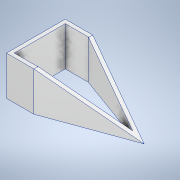
# Autodesk Inventor part: Wedge_wall
Saved by Autodesk Inventor 2020 (Build 240168000, 168)
## iProperties
Created: 2020-01-24
Part Number: Wedge_wall
Material: Aluminum 6061
Document SubType Name: Modeling
Designer: Connor
Density: 2.7 g/cm^3
Appearance: Aluminum - Flat
Mass: 1317.92 g
Surface Area: 1114.86 cm^2
Volume: 488.119 cm^3
Author: Connor
Autodesk Inventor part; units mm, degrees
ref_plane "YZ Plane" through (0, 0, 0) normal (1, 0, 0) x (0, 1, 0)
ref_plane "XZ Plane" through (0, 0, 0) normal (0, 1, 0) x (-1, 0, 0)
sketch "Sketch2" plane through (0, 0, 0) normal (0, 1, 0) x (-1, 0, 0)
  line L0 (0, 0) -> (150, 0)
  line L1 (150, 0) -> (150, -70.0962)
  line L2 (0, -70.0962) -> (0, 0)
  line L3 (102.7189, -200) -> (47.2811, -200)
  line L4 (102.7189, -200) -> (150, -70.0962)
  line L5 (47.2811, -200) -> (0, -70.0962)
  line L6 (0, -70.0962) -> (0, -200)
  line L7 (150, -70.0962) -> (150, -200)
  line L8 (0, -200) -> (150, -200)
  line L9 (102.7189, -200) -> (75, -276.157)
  line L10 (47.2811, -200) -> (75, -276.157)
  dimension "d7" = 150
  dimension "d23" = 70.0962
  dimension "d24" = 200
  dimension "d36" = 20
  dimension "d37" = 20
  constraints: 22 end point, 3 collinear, 3 horizontal, 3 vertical, 1 parallel, 1 perpendicular, 1 other
  measures "d7" distance of L0.start L0.end
  measures "d23" distance of L2.start L0.start
  measures "d24" distance of L6.end L0.start
  measures "d36" angle of L7 L4
  measures "d37" angle of L6 L5
extrude "Extrusion1" add sketch "Sketch2" along normal blind 100 contours L0 L1 L4 L3 L5 L2 | L3 L9 L10
sketch "Sketch11" plane through (0, 100, 0) normal (0, 1, 0) x (1, 0, 0)
  line L0 (0, 70.0962) -> (-75, 276.157) projected
  line L1 (-75, 276.157) -> (-150, 70.0962) projected
  line L2 (-150, 70.0962) -> (-150, 0) projected
  line L3 (-150, 0) -> (0, 0) projected
  line L4 (0, 0) -> (0, 70.0962) projected
  line L5 (-10, 68.3329) -> (-75, 246.919)
  line L6 (-75, 246.919) -> (-140, 68.3329)
  line L7 (-140, 68.3329) -> (-140, 10)
  line L8 (-140, 10) -> (-10, 10)
  line L9 (-10, 10) -> (-10, 68.3329)
  dimension "d46" = 10
  constraints: 10 end point, 4 other
  measures "d46" distance between parallel lines of L4 L9
extrude "Extrusion9" cut sketch "Sketch11" against normal blind 90 contours L9 L8 L7 L6 L5
ref_plane "Work Plane4" through (0, 100, -70.0962) normal (0, -0.8997, 0.4366) x (-1, 0, 0)
sketch "Sketch12" plane through (0, 100, -70.0962) normal (0, -0.8997, 0.4366) x (-1, 0, 0)
  line L0 (0, 0) -> (154.5136, 0)
  line L1 (154.5136, 0) -> (154.5136, 238.9342)
  line L2 (154.5136, 238.9342) -> (0, 238.9342)
  line L3 (0, 238.9342) -> (0, 0)
  point P0 (0, -19.4027)
  constraints: 8 end point, 2 parallel, 1 horizontal, 1 perpendicular
extrude "Extrusion10" cut sketch "Sketch12" against normal blind 90
sketch "Sketch13" plane through (0, 10, 0) normal (0, 1, 0) x (1, 0, 0)
  line L0 (-140, 10) -> (-140, 68.3329) projected
  line L1 (-10, 10) -> (-140, 10) projected
  line L2 (-10, 68.3329) -> (-10, 10) projected
  line L3 (-75, 246.919) -> (-10, 68.3329) projected
  line L4 (-140, 68.3329) -> (-75, 246.919) projected
  circle A0 centre (-75, 222.9149) radius 2.5
  line L5 (-75, 222.9149) -> (-10, 44.3288)
  line L6 (-75, 222.9149) -> (97.0532, 222.9149) construction
  line L7 (-75, 222.9149) -> (-140, 44.3288)
  circle A1 centre (-71.5798, 213.518) radius 2.5
  circle A2 centre (-68.1596, 204.121) radius 2.5
  circle A3 centre (-64.7394, 194.7241) radius 2.5
  circle A4 centre (-61.3192, 185.3272) radius 2.5
  circle A5 centre (-57.899, 175.9302) radius 2.5
  circle A6 centre (-54.4788, 166.5333) radius 2.5
  circle A7 centre (-51.0586, 157.1364) radius 2.5
  circle A8 centre (-47.6384, 147.7395) radius 2.5
  circle A9 centre (-44.2182, 138.3425) radius 2.5
  circle A10 centre (-40.798, 128.9456) radius 2.5
  circle A11 centre (-37.3778, 119.5487) radius 2.5
  circle A12 centre (-78.4202, 213.518) radius 2.5
  circle A13 centre (-75, 204.121) radius 2.5
  circle A14 centre (-71.5798, 194.7241) radius 2.5
  circle A15 centre (-68.1596, 185.3272) radius 2.5
  circle A16 centre (-64.7394, 175.9302) radius 2.5
  circle A17 centre (-61.3192, 166.5333) radius 2.5
  circle A18 centre (-57.899, 157.1364) radius 2.5
  circle A19 centre (-54.4788, 147.7395) radius 2.5
  circle A20 centre (-51.0586, 138.3425) radius 2.5
  circle A21 centre (-47.6384, 128.9456) radius 2.5
  circle A22 centre (-44.2182, 119.5487) radius 2.5
  circle A23 centre (-40.798, 110.1518) radius 2.5
  circle A24 centre (-81.8404, 204.121) radius 2.5
  circle A25 centre (-78.4202, 194.7241) radius 2.5
  circle A26 centre (-75, 185.3272) radius 2.5
  circle A27 centre (-71.5798, 175.9302) radius 2.5
  circle A28 centre (-68.1596, 166.5333) radius 2.5
  circle A29 centre (-64.7394, 157.1364) radius 2.5
  circle A30 centre (-61.3192, 147.7395) radius 2.5
  circle A31 centre (-57.899, 138.3425) radius 2.5
  circle A32 centre (-54.4788, 128.9456) radius 2.5
  circle A33 centre (-51.0586, 119.5487) radius 2.5
  circle A34 centre (-47.6384, 110.1518) radius 2.5
  circle A35 centre (-44.2182, 100.7548) radius 2.5
  circle A36 centre (-85.2606, 194.7241) radius 2.5
  circle A37 centre (-81.8404, 185.3272) radius 2.5
  circle A38 centre (-78.4202, 175.9302) radius 2.5
  circle A39 centre (-75, 166.5333) radius 2.5
  circle A40 centre (-71.5798, 157.1364) radius 2.5
  circle A41 centre (-68.1596, 147.7395) radius 2.5
  circle A42 centre (-64.7394, 138.3425) radius 2.5
  circle A43 centre (-61.3192, 128.9456) radius 2.5
  circle A44 centre (-57.899, 119.5487) radius 2.5
  circle A45 centre (-54.4788, 110.1518) radius 2.5
  circle A46 centre (-51.0586, 100.7548) radius 2.5
  circle A47 centre (-47.6384, 91.3579) radius 2.5
  circle A48 centre (-88.6808, 185.3272) radius 2.5
  circle A49 centre (-85.2606, 175.9302) radius 2.5
  circle A50 centre (-81.8404, 166.5333) radius 2.5
  circle A51 centre (-78.4202, 157.1364) radius 2.5
  circle A52 centre (-75, 147.7395) radius 2.5
  circle A53 centre (-71.5798, 138.3425) radius 2.5
  circle A54 centre (-68.1596, 128.9456) radius 2.5
  circle A55 centre (-64.7394, 119.5487) radius 2.5
  circle A56 centre (-61.3192, 110.1518) radius 2.5
  circle A57 centre (-57.899, 100.7548) radius 2.5
  circle A58 centre (-54.4788, 91.3579) radius 2.5
  circle A59 centre (-51.0586, 81.961) radius 2.5
  circle A60 centre (-92.101, 175.9302) radius 2.5
  circle A61 centre (-88.6808, 166.5333) radius 2.5
  circle A62 centre (-85.2606, 157.1364) radius 2.5
  circle A63 centre (-81.8404, 147.7395) radius 2.5
  circle A64 centre (-78.4202, 138.3425) radius 2.5
  circle A65 centre (-75, 128.9456) radius 2.5
  circle A66 centre (-71.5798, 119.5487) radius 2.5
  circle A67 centre (-68.1596, 110.1518) radius 2.5
  circle A68 centre (-64.7394, 100.7548) radius 2.5
  circle A69 centre (-61.3192, 91.3579) radius 2.5
  circle A70 centre (-57.899, 81.961) radius 2.5
  circle A71 centre (-54.4788, 72.5641) radius 2.5
  circle A72 centre (-95.5212, 166.5333) radius 2.5
  circle A73 centre (-92.101, 157.1364) radius 2.5
  circle A74 centre (-88.6808, 147.7395) radius 2.5
  circle A75 centre (-85.2606, 138.3425) radius 2.5
  circle A76 centre (-81.8404, 128.9456) radius 2.5
  circle A77 centre (-78.4202, 119.5487) radius 2.5
  circle A78 centre (-75, 110.1518) radius 2.5
  circle A79 centre (-71.5798, 100.7548) radius 2.5
  circle A80 centre (-68.1596, 91.3579) radius 2.5
  circle A81 centre (-64.7394, 81.961) radius 2.5
  circle A82 centre (-61.3192, 72.5641) radius 2.5
  circle A83 centre (-57.899, 63.1671) radius 2.5
  circle A84 centre (-98.9414, 157.1364) radius 2.5
  circle A85 centre (-95.5212, 147.7395) radius 2.5
  circle A86 centre (-92.101, 138.3425) radius 2.5
  circle A87 centre (-88.6808, 128.9456) radius 2.5
  circle A88 centre (-85.2606, 119.5487) radius 2.5
  circle A89 centre (-81.8404, 110.1518) radius 2.5
  circle A90 centre (-78.4202, 100.7548) radius 2.5
  circle A91 centre (-75, 91.3579) radius 2.5
  circle A92 centre (-71.5798, 81.961) radius 2.5
  circle A93 centre (-68.1596, 72.5641) radius 2.5
  circle A94 centre (-64.7394, 63.1671) radius 2.5
  circle A95 centre (-61.3192, 53.7702) radius 2.5
  circle A96 centre (-102.3616, 147.7395) radius 2.5
  circle A97 centre (-98.9414, 138.3425) radius 2.5
  circle A98 centre (-95.5212, 128.9456) radius 2.5
  circle A99 centre (-92.101, 119.5487) radius 2.5
  circle A100 centre (-88.6808, 110.1518) radius 2.5
  circle A101 centre (-85.2606, 100.7548) radius 2.5
  circle A102 centre (-81.8404, 91.3579) radius 2.5
  circle A103 centre (-78.4202, 81.961) radius 2.5
  circle A104 centre (-75, 72.5641) radius 2.5
  circle A105 centre (-71.5798, 63.1671) radius 2.5
  circle A106 centre (-68.1596, 53.7702) radius 2.5
  circle A107 centre (-64.7394, 44.3733) radius 2.5
  circle A108 centre (-105.7818, 138.3425) radius 2.5
  circle A109 centre (-102.3616, 128.9456) radius 2.5
  circle A110 centre (-98.9414, 119.5487) radius 2.5
  circle A111 centre (-95.5212, 110.1518) radius 2.5
  circle A112 centre (-92.101, 100.7548) radius 2.5
  circle A113 centre (-88.6808, 91.3579) radius 2.5
  circle A114 centre (-85.2606, 81.961) radius 2.5
  circle A115 centre (-81.8404, 72.5641) radius 2.5
  circle A116 centre (-78.4202, 63.1671) radius 2.5
  circle A117 centre (-75, 53.7702) radius 2.5
  circle A118 centre (-71.5798, 44.3733) radius 2.5
  circle A119 centre (-68.1596, 34.9764) radius 2.5
  circle A120 centre (-109.202, 128.9456) radius 2.5
  circle A121 centre (-105.7818, 119.5487) radius 2.5
  circle A122 centre (-102.3616, 110.1518) radius 2.5
  circle A123 centre (-98.9414, 100.7548) radius 2.5
  circle A124 centre (-95.5212, 91.3579) radius 2.5
  circle A125 centre (-92.101, 81.961) radius 2.5
  circle A126 centre (-88.6808, 72.5641) radius 2.5
  circle A127 centre (-85.2606, 63.1671) radius 2.5
  circle A128 centre (-81.8404, 53.7702) radius 2.5
  circle A129 centre (-78.4202, 44.3733) radius 2.5
  circle A130 centre (-75, 34.9764) radius 2.5
  circle A131 centre (-71.5798, 25.5794) radius 2.5
  circle A132 centre (-112.6222, 119.5487) radius 2.5
  circle A133 centre (-109.202, 110.1518) radius 2.5
  circle A134 centre (-105.7818, 100.7548) radius 2.5
  circle A135 centre (-102.3616, 91.3579) radius 2.5
  circle A136 centre (-98.9414, 81.961) radius 2.5
  circle A137 centre (-95.5212, 72.5641) radius 2.5
  circle A138 centre (-92.101, 63.1671) radius 2.5
  circle A139 centre (-88.6808, 53.7702) radius 2.5
  circle A140 centre (-85.2606, 44.3733) radius 2.5
  circle A141 centre (-81.8404, 34.9764) radius 2.5
  circle A142 centre (-78.4202, 25.5794) radius 2.5
  circle A143 centre (-75, 16.1825) radius 2.5
  point P0 (0, 0)
  dimension "d51" = 5
  dimension "d52" = 70
  dimension "d53" = 70
  dimension "d56" = 10
  dimension "d59" = 10
  constraints: 144 centre point, 6 end point, 2 point on line, 1 horizontal, 288 other
  measures "d51" diameter of A0
  measures "d52" angle of L5 L6
  measures "d53" angle of L6 L7
  measures "d56" distance of L5.start A1.centre
  measures "d59" distance of L5.start A12.centre
extrude "Extrusion11" cut sketch "Sketch13" against normal through all contours A132 L7 | L7 A132 | A11 L5 | L5 A11 | A120 L7 | L7 A120 | A10 L5 | L5 A10 | A108 L7 | L7 A108 | A9 L5 | L5 A9 | A96 L7 | L7 A96 | A8 L5 | L5 A8 | A84 L7 | L7 A84 | A7 L5 | L5 A7 | A72 L7 | L7 A72 | A6 L5 | L5 A6 | A60 L7 | L7 A60 | A5 L5 | L5 A5 | A48 L7 | L7 A48 | A4 L5 | L5 A4 | A36 L7 | L7 A36 | A3 L5 | L5 A3 | A24 L7 | L7 A24 | A2 L5 | L5 A2 | A12 L7 | L7 A12 | A1 L5 | L5 A1 | L7 L5 A0 | A0 L5 L7 | A13 | A14 | A15 | A16 | A17 | A18 | A19 | A20 | A21 | A22 | A23 | A25 | A26 | A27 | A28 | A29 | A30 | A31 | A32 | A33 | A34 | A35 | A37 | A38 | A39 | A40 | A41 | A42 | A43 | A44 | A45 | A46 | A47 | A49 | A50 | A51 | A52 | A53 | A54 | A55 | A56 | A57 | A58 | A59 | A61 | A62 | A63 | A64 | A65 | A66 | A67 | A68 | A69 | A70 | A71 | A73 | A74 | A75 | A76 | A77 | A78 | A79 | A80 | A81 | A82 | A83 | A85 | A86 | A87 | A88 | A89 | A90 | A91 | A92 | A93 | A94 | A95 | A97 | A98 | A99 | A100 | A101 | A102 | A103 | A104 | A105 | A107 | A109 | A110 | A111 | A112 | A113 | A114 | A115 | A116 | A117 | A118 | A119 | A121 | A122 | A123 | A124 | A125 | A126 | A127 | A128 | A129 | A130 | A131 | A133 | A134 | A135 | A136 | A137 | A138 | A139 | A140 | A141 | A142 | A143
sketch "Sketch15" plane through (0, 10, 0) normal (0, 1, 0) x (1, 0, 0)
  circle A0 centre (-68.1596, 204.121) radius 2.5 projected
  circle A1 centre (-78.4202, 213.518) radius 2.5 projected
  circle A2 centre (-92.101, 175.9302) radius 2.5 projected
  circle A3 centre (-71.5798, 175.9302) radius 2.5 projected
  circle A4 centre (-68.1596, 185.3272) radius 2.5 projected
  circle A5 centre (-95.5212, 128.9456) radius 2.5 projected
  circle A6 centre (-92.101, 157.1364) radius 2.5 projected
  circle A7 centre (-92.101, 138.3425) radius 2.5 projected
  circle A8 centre (-102.3616, 147.7395) radius 2.5 projected
  circle A9 centre (-57.899, 157.1364) radius 2.5 projected
  circle A10 centre (-61.3192, 147.7395) radius 2.5 projected
  circle A11 centre (-71.5798, 157.1364) radius 2.5 projected
  circle A12 centre (-81.8404, 166.5333) radius 2.5 projected
  circle A13 centre (-68.1596, 128.9456) radius 2.5 projected
  circle A14 centre (-81.8404, 128.9456) radius 2.5 projected
  circle A15 centre (-85.2606, 100.7548) radius 2.5 projected
  circle A16 centre (-88.6808, 91.3579) radius 2.5 projected
  circle A17 centre (-92.101, 81.961) radius 2.5 projected
  circle A18 centre (-105.7818, 100.7548) radius 2.5 projected
  circle A19 centre (-112.6222, 119.5487) radius 2.5 projected
  circle A20 centre (-54.4788, 110.1518) radius 2.5 projected
  circle A21 centre (-54.4788, 91.3579) radius 2.5 projected
  circle A22 centre (-61.3192, 91.3579) radius 2.5 projected
  circle A23 centre (-71.5798, 100.7548) radius 2.5 projected
  circle A24 centre (-78.4202, 100.7548) radius 2.5 projected
  circle A25 centre (-75, 34.9764) radius 2.5 projected
  circle A26 centre (-75, 16.1825) radius 2.5 projected
  circle A27 centre (-54.4788, 72.5641) radius 2.5 projected
  circle A28 centre (-78.4202, 63.1671) radius 2.5 projected
  circle A29 centre (-95.5212, 72.5641) radius 2.5 projected
  circle A30 centre (-75, 53.7702) radius 2.5 projected
  circle A31 centre (-75, 72.5641) radius 2.5 projected
  circle A32 centre (-44.2182, 138.3425) radius 2.5 projected
  circle A33 centre (-47.6384, 91.3579) radius 2.5 projected
  circle A34 centre (-51.0586, 119.5487) radius 2.5 projected
  circle A35 centre (-51.0586, 138.3425) radius 2.5 projected
  circle A36 centre (-40.798, 110.1518) radius 2.5 projected
  circle A37 centre (-51.0586, 100.7548) radius 2.5 projected
  circle A38 centre (-40.798, 128.9456) radius 2.5 projected
  circle A39 centre (-61.3192, 53.7702) radius 2.5 projected
  circle A40 centre (-81.8404, 72.5641) radius 2.5 projected
  circle A41 centre (-88.6808, 53.7702) radius 2.5 projected
  circle A42 centre (-71.5798, 44.3733) radius 2.5 projected
  circle A43 centre (-64.7394, 63.1671) radius 2.5 projected
  circle A44 centre (-68.1596, 72.5641) radius 2.5 projected
  circle A45 centre (-71.5798, 25.5794) radius 2.5 projected
  circle A46 centre (-75, 91.3579) radius 2.5 projected
  circle A47 centre (-68.1596, 91.3579) radius 2.5 projected
  circle A48 centre (-57.899, 81.961) radius 2.5 projected
  circle A49 centre (-71.5798, 119.5487) radius 2.5 projected
  circle A50 centre (-64.7394, 119.5487) radius 2.5 projected
  circle A51 centre (-81.8404, 91.3579) radius 2.5 projected
  circle A52 centre (-95.5212, 91.3579) radius 2.5 projected
  circle A53 centre (-109.202, 110.1518) radius 2.5 projected
  circle A54 centre (-85.2606, 81.961) radius 2.5 projected
  circle A55 centre (-98.9414, 119.5487) radius 2.5 projected
  circle A56 centre (-54.4788, 166.5333) radius 2.5 projected
  circle A57 centre (-81.8404, 147.7395) radius 2.5 projected
  circle A58 centre (-78.4202, 157.1364) radius 2.5 projected
  circle A59 centre (-68.1596, 147.7395) radius 2.5 projected
  circle A60 centre (-57.899, 138.3425) radius 2.5 projected
  circle A61 centre (-54.4788, 147.7395) radius 2.5 projected
  circle A62 centre (-98.9414, 157.1364) radius 2.5 projected
  circle A63 centre (-88.6808, 128.9456) radius 2.5 projected
  circle A64 centre (-88.6808, 147.7395) radius 2.5 projected
  circle A65 centre (-102.3616, 128.9456) radius 2.5 projected
  circle A66 centre (-71.5798, 194.7241) radius 2.5 projected
  circle A67 centre (-75, 185.3272) radius 2.5 projected
  circle A68 centre (-85.2606, 175.9302) radius 2.5 projected
  circle A69 centre (-81.8404, 204.121) radius 2.5 projected
  circle A70 centre (-64.7394, 194.7241) radius 2.5 projected
  circle A71 centre (-71.5798, 213.518) radius 2.5 projected
  circle A72 centre (-57.899, 175.9302) radius 2.5 projected
  circle A73 centre (-88.6808, 185.3272) radius 2.5 projected
  circle A74 centre (-81.8404, 185.3272) radius 2.5 projected
  circle A75 centre (-64.7394, 175.9302) radius 2.5 projected
  circle A76 centre (-98.9414, 138.3425) radius 2.5 projected
  circle A77 centre (-85.2606, 157.1364) radius 2.5 projected
  circle A78 centre (-95.5212, 147.7395) radius 2.5 projected
  circle A79 centre (-105.7818, 138.3425) radius 2.5 projected
  circle A80 centre (-61.3192, 166.5333) radius 2.5 projected
  circle A81 centre (-64.7394, 157.1364) radius 2.5 projected
  circle A82 centre (-75, 166.5333) radius 2.5 projected
  circle A83 centre (-61.3192, 128.9456) radius 2.5 projected
  circle A84 centre (-71.5798, 138.3425) radius 2.5 projected
  circle A85 centre (-75, 128.9456) radius 2.5 projected
  circle A86 centre (-88.6808, 110.1518) radius 2.5 projected
  circle A87 centre (-92.101, 100.7548) radius 2.5 projected
  circle A88 centre (-98.9414, 100.7548) radius 2.5 projected
  circle A89 centre (-98.9414, 81.961) radius 2.5 projected
  circle A90 centre (-85.2606, 119.5487) radius 2.5 projected
  circle A91 centre (-57.899, 119.5487) radius 2.5 projected
  circle A92 centre (-57.899, 100.7548) radius 2.5 projected
  circle A93 centre (-64.7394, 100.7548) radius 2.5 projected
  circle A94 centre (-75, 110.1518) radius 2.5 projected
  circle A95 centre (-81.8404, 110.1518) radius 2.5 projected
  circle A96 centre (-68.1596, 34.9764) radius 2.5 projected
  circle A97 centre (-78.4202, 25.5794) radius 2.5 projected
  circle A98 centre (-61.3192, 72.5641) radius 2.5 projected
  circle A99 centre (-85.2606, 44.3733) radius 2.5 projected
  circle A100 centre (-81.8404, 53.7702) radius 2.5 projected
  circle A101 centre (-85.2606, 63.1671) radius 2.5 projected
  circle A102 centre (-71.5798, 63.1671) radius 2.5 projected
  circle A103 centre (-47.6384, 147.7395) radius 2.5 projected
  circle A104 centre (-51.0586, 81.961) radius 2.5 projected
  circle A105 centre (-47.6384, 110.1518) radius 2.5 projected
  circle A106 centre (-47.6384, 128.9456) radius 2.5 projected
  circle A107 centre (-44.2182, 119.5487) radius 2.5 projected
  circle A108 centre (-44.2182, 100.7548) radius 2.5 projected
  circle A109 centre (-37.3778, 119.5487) radius 2.5 projected
  circle A110 centre (-51.0586, 157.1364) radius 2.5 projected
  circle A111 centre (-64.7394, 44.3733) radius 2.5 projected
  circle A112 centre (-78.4202, 44.3733) radius 2.5 projected
  circle A113 centre (-88.6808, 72.5641) radius 2.5 projected
  circle A114 centre (-92.101, 63.1671) radius 2.5 projected
  circle A115 centre (-57.899, 63.1671) radius 2.5 projected
  circle A116 centre (-81.8404, 34.9764) radius 2.5 projected
  circle A117 centre (-71.5798, 81.961) radius 2.5 projected
  circle A118 centre (-64.7394, 81.961) radius 2.5 projected
  circle A119 centre (-78.4202, 119.5487) radius 2.5 projected
  circle A120 centre (-68.1596, 110.1518) radius 2.5 projected
  circle A121 centre (-61.3192, 110.1518) radius 2.5 projected
  circle A122 centre (-78.4202, 81.961) radius 2.5 projected
  circle A123 centre (-102.3616, 110.1518) radius 2.5 projected
  circle A124 centre (-102.3616, 91.3579) radius 2.5 projected
  circle A125 centre (-105.7818, 119.5487) radius 2.5 projected
  circle A126 centre (-95.5212, 110.1518) radius 2.5 projected
  circle A127 centre (-92.101, 119.5487) radius 2.5 projected
  circle A128 centre (-78.4202, 138.3425) radius 2.5 projected
  circle A129 centre (-75, 147.7395) radius 2.5 projected
  circle A130 centre (-64.7394, 138.3425) radius 2.5 projected
  circle A131 centre (-54.4788, 128.9456) radius 2.5 projected
  circle A132 centre (-68.1596, 166.5333) radius 2.5 projected
  circle A133 centre (-95.5212, 166.5333) radius 2.5 projected
  circle A134 centre (-109.202, 128.9456) radius 2.5 projected
  circle A135 centre (-85.2606, 138.3425) radius 2.5 projected
  circle A136 centre (-88.6808, 166.5333) radius 2.5 projected
  circle A137 centre (-75, 204.121) radius 2.5 projected
  circle A138 centre (-78.4202, 194.7241) radius 2.5 projected
  circle A139 centre (-78.4202, 175.9302) radius 2.5 projected
  circle A140 centre (-85.2606, 194.7241) radius 2.5 projected
  circle A141 centre (-61.3192, 185.3272) radius 2.5 projected
  circle A142 centre (-75, 222.9149) radius 2.5 projected
  line L0 (-140, 10) -> (-140, 68.3329) projected
  line L1 (-10, 10) -> (-140, 10) projected
  line L2 (-10, 68.3329) -> (-10, 10) projected
  line L3 (-75, 246.919) -> (-10, 68.3329) projected
  line L4 (-140, 68.3329) -> (-75, 246.919) projected
  point P0 (0, 0)
extrude "Extrusion13" cut sketch "Sketch15" against normal blind 90
body "Solid1"
